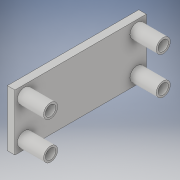
# Autodesk Inventor part: Part9
Saved by Autodesk Inventor 2019 (Build 230136000, 136)
## iProperties
Created: 2021-08-30
Part Number: Part9
Material: 一般
Document SubType Name: Sheet Metal
Designer: yuta
Density: 1 g/cm^3
Sheet Metal Rule: Default_mm
Appearance: 既定
Author: yuta
Autodesk Inventor part; units mm, degrees
ref_plane "YZ Plane" through (0, 0, 0) normal (1, 0, 0) x (0, 1, 0)
ref_plane "XZ Plane" through (0, 0, 0) normal (0, 1, 0) x (-1, 0, 0)
ref_plane "XY Plane" through (0, 0, 0) normal (0, 0, 1) x (1, 0, 0)
sketch "スケッチ1" plane through (0, 0, 0) normal (1, 0, 0) x (0, 1, 0)
  line L0 (30.947, 69.6362) -> (-29.053, 69.6362)
  line L1 (-29.053, 69.6362) -> (-29.053, -70.3638)
  line L2 (-29.053, -70.3638) -> (30.947, -70.3638)
  line L3 (30.947, -70.3638) -> (30.947, 69.6362)
  point P0 (0, 0)
  dimension "d0" = 60
  dimension "d1" = 140
  constraints: 8 end point, 2 parallel, 1 horizontal, 1 perpendicular
  measures "d0" distance of L2.end L1.end
  measures "d1" distance of L1.end L0.end
extrude "押し出し1" add sketch "スケッチ1" along normal blind 8.1
sketch "スケッチ2" plane through (8.1, 0, 0) normal (1, 0, 0) x (0, 0, -1)
  circle A0 centre (-59.6362, 20.947) radius 7.5
  line L0 (70.3638, 30.947) -> (-69.6362, 30.947) projected
  line L1 (-69.6362, 30.947) -> (-69.6362, -29.053) projected
  circle A1 centre (-59.6362, -19.053) radius 7.5
  line L2 (-69.6362, -29.053) -> (70.3638, -29.053) projected
  circle A2 centre (60.3638, 20.947) radius 7.5
  line L3 (70.3638, -29.053) -> (70.3638, 30.947) projected
  circle A3 centre (60.3638, -19.053) radius 7.5
  circle A4 centre (-59.6362, 20.947) radius 5.5
  circle A5 centre (-59.6362, -19.053) radius 5.5
  circle A6 centre (60.3638, 20.947) radius 5.5
  circle A7 centre (60.3638, -19.053) radius 5.5
  point P0 (0, 0)
  dimension "d4" = 15
  dimension "d5" = 10
  dimension "d6" = 10
  dimension "d7" = 15
  dimension "d8" = 10
  dimension "d9" = 15
  dimension "d10" = 10
  dimension "d11" = 15
  dimension "d12" = 11
  dimension "d13" = 11
  dimension "d14" = 11
  dimension "d15" = 11
  constraints: 8 centre point, 4 coincident
  measures "d4" diameter of A0
  measures "d5" distance from line of A0.centre L0
  measures "d6" distance from line of L1 A0.centre
  measures "d7" diameter of A1
  measures "d8" distance from line of L2 A1.centre
  measures "d9" diameter of A2
  measures "d10" distance from line of L3 A2.centre
  measures "d11" diameter of A3
  measures "d12" diameter of A4
  measures "d13" diameter of A5
  measures "d14" diameter of A6
  measures "d15" diameter of A7
extrude "押し出し2" add sketch "スケッチ2" along normal blind 28 contours A0 | A1 | A2 | A3
equation "\"BendRadius\" = Thickness"
equation "\"BendReliefWidth\" = Thickness"
equation "\"BendReliefDepth\" = 0.5 * Thickness"
equation "\"CornerReliefSize\" = 4 * Thickness"
equation "\"MinimumRemnant\" = 2 * Thickness"
equation "\"TransitionRadius\" = BendRadius"
equation "\"JacobiRadiusSize\" = BendRadius"
equation "\"GapSize\" = Thickness"
equation "\"Thickness\" = 0.5"
